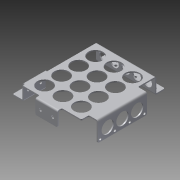
# Autodesk Inventor part: Chassis Battery Mount Part1
Saved by Autodesk Inventor 2013 (Build 170138000, 138)
## iProperties
Created: 2013-01-24
Part Number: Chassis Battery Mount Part1
Material: Aluminum 6061
Document SubType Name: Sheet Metal
Designer: Moses
Density: 2.71 g/cm^3
Sheet Metal Rule: Default
Mass: 289.922 g
Surface Area: 784.778 cm^2
Volume: 106.982 cm^3
Flat Pattern Width: 28.8793 cm
Flat Pattern Length: 29.5143 cm
Flat Pattern Area: 852.352 cm^2
Sheet Metal Width: 11.370 in
Sheet Metal Length: 11.620 in
Sheet Metal Area: 132.115 in^2
Author: Moses
Autodesk Inventor part; units mm, degrees
ref_plane "YZ Plane" through (0, 0, 0) normal (1, 0, 0) x (0, 1, 0)
ref_plane "XZ Plane" through (0, 0, 0) normal (0, 1, 0) x (-1, 0, 0)
ref_plane "XY Plane" through (0, 0, 0) normal (0, 0, 1) x (1, 0, 0)
sketch "Sketch1" plane through (0, 0, 0) normal (0, 1, 0) x (-1, 0, 0)
  line L0 (0, 0) -> (152.4, 0)
  line L1 (152.4, 0) -> (152.4, 25.4)
  line L2 (152.4, 25.4) -> (0, 25.4)
  line L3 (0, 25.4) -> (0, 0)
  line L4 (0, 12.7) -> (152.4, 12.7) construction
  circle A0 centre (12.7, 12.7) radius 3.302
  circle A1 centre (38.1, 12.7) radius 3.302
  circle A2 centre (63.5, 12.7) radius 3.302
  circle A3 centre (88.9, 12.7) radius 3.302
  circle A4 centre (114.3, 12.7) radius 3.302
  circle A5 centre (139.7, 12.7) radius 3.302
  dimension "d0" = 25.4
  dimension "d1" = 152.4
  dimension "d2" = 6.604
  dimension "d3" = 12.7
  dimension "d6" = 25.4
  dimension "d11" = 12.7
  measures "d0" distance of L2.end L0.start
  measures "d1" distance of L0.start L0.end
  measures "d2" diameter of A0
  measures "d3" distance from line of A0.centre L3
  measures "d6" distance of A0.centre A1.centre
  measures "d11" distance from line of L1 A5.centre
extrude "Plate1" add sketch "Sketch1" along normal blind 3.175
sketch "Sketch2" plane through (0, 0, 22.225) normal (0, 0, 1) x (1, 0, 0)
  line L0 (-152.4, 0) -> (0, 0)
  line L1 (0, 0) -> (0, 38.1)
  line L2 (0, 38.1) -> (-152.4, 38.1)
  line L3 (-152.4, 38.1) -> (-152.4, 0)
  constraints: 6 end point, 1 horizontal, 1 perpendicular, 1 vertical
edge flange "Flange1" height 38.1 angle 90 thickness 3.175 bend radius 1.27 thickness toward (0, 0, 1) relief straight relief width 3.175 relief depth 1.5875 edges at (-76.2, 3.175, 25.4) wall of the first edge with corners at (-152.4, 0, 22.225) (0, 0, 22.225) (0, 38.1, 22.225) (-152.4, 38.1, 22.225)
bend "Bend1"
corner "Corner1"
sketch "Sketch3" plane through (-152.4, 38.1, 25.4) normal (0, 1, 0) x (-1, 0, 0)
  line L0 (-152.4, 0) -> (0, 0)
  line L1 (0, 0) -> (0, 190.5)
  line L2 (0, 190.5) -> (-152.4, 190.5)
  line L3 (-152.4, 190.5) -> (-152.4, 0)
  constraints: 6 end point, 1 horizontal, 1 perpendicular, 1 vertical
edge flange "Flange2" height 193.675 angle 90 thickness 3.175 bend radius 1.27 thickness toward (0, 1, 0) relief straight relief width 3.175 relief depth 1.5875 edges at (-76.2, 38.1, 25.4) wall of the first edge with corners at (0, 38.1, 25.4) (-152.4, 38.1, 25.4) (-152.4, 38.1, 215.9) (0, 38.1, 215.9)
bend "Bend2"
corner "Corner2"
sketch "Sketch4" plane through (-152.4, 41.275, 215.9) normal (0, 1, 0) x (1, 0, 0)
  line L0 (0, 0) -> (0, 189.23) projected
  line L1 (152.4, 189.23) -> (152.4, 0) projected
  line L2 (-6.35, 6.35) -> (-6.35, 63.5)
  line L3 (-6.35, 63.5) -> (0, 63.5)
  line L4 (152.4, 189.23) -> (0, 189.23) projected
  line L5 (152.4, 0) -> (0, 0) projected
  circle A0 centre (28.575, 28.575) radius 19.05
  circle A1 centre (28.575, 72.6017) radius 19.05
  circle A2 centre (28.575, 116.6283) radius 19.05
  circle A3 centre (28.575, 160.655) radius 19.05
  circle A4 centre (76.2, 28.575) radius 19.05
  circle A5 centre (76.2, 72.6017) radius 19.05
  circle A6 centre (76.2, 116.6283) radius 19.05
  circle A7 centre (76.2, 160.655) radius 19.05
  circle A8 centre (123.825, 28.575) radius 19.05
  circle A9 centre (123.825, 72.6017) radius 19.05
  circle A10 centre (123.825, 116.6283) radius 19.05
  circle A11 centre (123.825, 160.655) radius 19.05
  line L6 (171.45, 19.05) -> (171.45, 146.05)
  line L7 (171.45, 146.05) -> (152.4, 146.05)
  line L8 (101.6, 0) -> (101.6, -6.35)
  line L9 (101.6, -6.35) -> (44.45, -6.35)
  line L10 (44.45, -6.35) -> (44.45, 0)
  line L11 (152.4, 19.05) -> (171.45, 19.05)
  line L12 (-6.35, 6.35) -> (0, 6.35)
  point P0 (152.4, 215.9)
  dimension "d33" = 57.15
  dimension "d35" = 6.35
  dimension "d64" = 38.1
  dimension "d65" = 28.575
  dimension "d66" = 28.575
  dimension "d69" = 44.0267
  dimension "d72" = 47.625
  dimension "d75" = 28.575
  dimension "d76" = 28.575
  dimension "d95" = 127
  dimension "d106" = 6.35
  dimension "d107" = 57.15
  dimension "d108" = 50.8
  dimension "d119" = 19.05
  dimension "d120" = 19.05
  dimension "d121" = 6.35
  dimension "d146" = 189.23
  constraints: 18 end point, 12 centre point, 6 perpendicular, 6 point on line, 2 horizontal, 2 vertical, 1 parallel, 22 other
  measures "d33" distance of L2.start L2.end
  measures "d35" distance of L2.end L3.end
  measures "d64" diameter of A0
  measures "d65" distance from line of L0 A0.centre
  measures "d66" distance from line of L5 A0.centre
  measures "d69" distance of A0.centre A1.centre
  measures "d72" distance of A0.centre A4.centre
  measures "d75" distance from line of L1 A8.centre
  measures "d76" distance from line of L4 A3.centre
  measures "d95" distance of L6.start L6.end
  measures "d106" distance of L9.end L10.end
  measures "d107" distance of L8.end L9.end
  measures "d108" distance from line of L1.end L8
  measures "d119" distance of L11.start L6.start
  measures "d120" distance from line of L1.end L11
  measures "d121" distance between parallel lines of L5 L12
  measures "d146" distance of L0.start L0.end
sheet face with bend "Face2" sketch "Sketch4" thickness 3.175 toward (0, -1, 0) bend radius 3.175 relief straight relief width 3.175 relief depth 1.5875 contours L12 L2 L3 L0 | L5 L8 L9 L10 | L1 L7 L6 L11
bend "Bend3"
sketch "Sketch5" plane through (-155.575, 41.275, 152.4) normal (-1, 0, 0) x (0, -1, 0)
  line L0 (0, 57.15) -> (0, 0)
  line L1 (0, 0) -> (41.275, 0)
  line L2 (41.275, 0) -> (41.275, 57.15)
  line L3 (41.275, 57.15) -> (0, 57.15)
  constraints: 6 end point, 1 horizontal, 1 perpendicular, 1 vertical
edge flange "Flange3" height 41.275 angle 90 thickness 3.175 bend radius 1.27 thickness toward (-1, 0, 0) relief straight relief width 3.175 relief depth 1.5875 edges at (-158.75, 38.1, 180.975) wall of the first edge with corners at (-155.575, 41.275, 209.55) (-155.575, 41.275, 152.4) (-155.575, 0, 152.4) (-155.575, 0, 209.55)
bend "Bend4"
corner "Corner3"
sketch "Sketch6" plane through (-155.575, 3.175, 209.55) normal (0, -1, 0) x (1, 0, 0)
  line L0 (0, -57.15) -> (0, 0)
  line L1 (0, 0) -> (-28.575, 0)
  line L2 (-28.575, 0) -> (-28.575, -57.15)
  line L3 (-28.575, -57.15) -> (0, -57.15)
  constraints: 6 end point, 1 horizontal, 1 perpendicular, 1 vertical
edge flange "Flange4" height 28.575 angle 90 thickness 3.175 bend radius 1.27 thickness toward (0, -1, 0) relief straight relief width 3.175 relief depth 1.5875 edges at (-158.75, 0, 180.975) wall of the first edge with corners at (-155.575, 3.175, 152.4) (-155.575, 3.175, 209.55) (-184.15, 3.175, 209.55) (-184.15, 3.175, 152.4)
bend "Bend5"
corner "Corner4"
sketch "Sketch7" plane through (-184.15, 3.175, 209.55) normal (0, 1, 0) x (1, 0, 0)
  circle A0 centre (12.7, 19.05) radius 3.302 projected
  circle A1 centre (12.7, 38.1) radius 3.302 projected
  point P0 (184.15, 209.55)
extrude "Cut1" cut sketch "Sketch7" against normal blind 3.175
fillet "Corner Round1" radius 3.175 10 edges at (-184.15, 1.5875, 209.55) (-184.15, 1.5875, 152.4) (-152.4, 1.5875, 0) (0, 1.5875, 0) (0, 39.6875, 69.85) (0, 39.6875, 196.85) (-50.8, 39.6875, 215.9) (-107.95, 39.6875, 215.9) (0, 39.6875, 215.9) (-152.4, 39.6875, 215.9)
extrude "Cut2" cut sketch "Sketch4" against normal blind 3.175 contours A0 | A1 | A2 | A3 | A4 | A5 | A6 | A7 | A8 | A9 | A10 | A11
sketch "Sketch8" plane through (0, 4.445, 22.225) normal (0, 0, -1) x (-1, 0, 0)
  line L0 (0, 32.385) -> (0, 0) projected
  line L1 (152.4, 32.385) -> (152.4, 0) projected
  line L2 (0, 16.1925) -> (152.4, 16.1925) construction
  circle A0 centre (19.05, 16.1925) radius 11.1125
  circle A1 centre (47.625, 16.1925) radius 11.1125
  circle A2 centre (76.2, 16.1925) radius 11.1125
  circle A3 centre (104.775, 16.1925) radius 11.1125
  circle A4 centre (133.35, 16.1925) radius 11.1125
  point P0 (0, -4.445)
  dimension "d79" = 22.225
  dimension "d83" = 19.05
  dimension "d84" = 152.4
  dimension "d87" = 28.575
  constraints: 5 centre point, 2 end point, 2 midpoint, 1 horizontal, 1 point on line, 8 other
  measures "d79" diameter of A0
  measures "d83" distance from line of A0.centre L0
  measures "d84" distance of L1.start L0.start
  measures "d87" distance of A0.centre A1.centre
extrude "Cut3" cut sketch "Sketch8" against normal blind 3.175
sketch "Sketch9" plane through (20.32, 36.83, 196.85) normal (1, 0, 0) x (0, 1, 0)
  line L0 (0, -127) -> (0, 0)
  line L1 (0, 0) -> (-46.355, 0)
  line L2 (-46.355, 0) -> (-46.355, -127)
  line L3 (-46.355, -127) -> (0, -127)
  constraints: 6 end point, 1 horizontal, 1 perpendicular, 1 vertical
edge flange "Flange5" height 50.8 angle 90 thickness 3.175 bend radius 1.27 thickness toward (1, 0, 0) relief straight relief width 3.175 relief depth 1.5875 edges at (19.05, 38.1, 133.35) wall of the first edge with corners at (20.32, 36.83, 69.85) (20.32, 36.83, 196.85) (20.32, -9.525, 196.85) (20.32, -9.525, 69.85)
bend "Bend6"
corner "Corner5"
sketch "Sketch10" plane through (-107.95, 36.83, 223.52) normal (0, 0, 1) x (1, 0, 0)
  line L0 (57.15, 0) -> (0, 0)
  line L1 (0, 0) -> (0, -33.655)
  line L2 (0, -33.655) -> (57.15, -33.655)
  line L3 (57.15, -33.655) -> (57.15, 0)
  constraints: 6 end point, 1 horizontal, 1 perpendicular, 1 vertical
edge flange "Flange6" height 38.1 angle 90 thickness 3.175 bend radius 1.27 thickness toward (0, 0, 1) relief straight relief width 3.175 relief depth 1.5875 edges at (-79.375, 38.1, 222.25) wall of the first edge with corners at (-50.8, 36.83, 223.52) (-107.95, 36.83, 223.52) (-107.95, 3.175, 223.52) (-50.8, 3.175, 223.52)
bend "Bend7"
corner "Corner6"
sketch "Sketch11" plane through (23.495, -9.525, 196.85) normal (1, 0, 0) x (0, 0, -1)
  line L0 (0, 0) -> (0, 46.355) projected
  line L1 (127, 0) -> (0, 0) projected
  line L2 (127, 46.355) -> (127, 0) projected
  line L3 (0, 23.1775) -> (127, 23.1775) construction
  circle A0 centre (25.4, 23.1775) radius 15.875
  circle A1 centre (63.5, 23.1775) radius 15.875
  circle A2 centre (101.6, 23.1775) radius 15.875
  line L4 (0, 6.35) -> (127, 6.35) construction
  circle A3 centre (6.35, 6.35) radius 3.302
  circle A4 centre (44.45, 6.35) radius 3.302
  circle A5 centre (82.55, 6.35) radius 3.302
  circle A6 centre (120.65, 6.35) radius 3.302
  point P0 (196.85, 9.525)
  dimension "d122" = 127
  dimension "d123" = 31.75
  dimension "d124" = 25.4
  dimension "d127" = 38.1
  dimension "d132" = 25.4
  dimension "d133" = 6.35
  dimension "d134" = 6.604
  dimension "d135" = 6.35
  dimension "d138" = 38.1
  dimension "d143" = 6.35
  constraints: 7 centre point, 4 end point, 4 point on line, 2 horizontal, 2 midpoint, 1 perpendicular, 10 other
  measures "d122" distance of L2.start L0.end
  measures "d123" diameter of A0
  measures "d124" distance from line of A0.centre L0
  measures "d127" distance of A0.centre A1.centre
  measures "d132" distance from line of L2 A2.centre
  measures "d133" distance between parallel lines of L1 L4
  measures "d134" diameter of A3
  measures "d135" distance from line of A3.centre L0
  measures "d138" distance of A3.centre A4.centre
  measures "d143" distance from line of L2 A6.centre
extrude "Cut4" cut sketch "Sketch11" against normal blind 3.175
sketch "Sketch12" plane through (-158.75, 36.83, 152.4) normal (-1, 0, 0) x (0, 0, 1)
  line L0 (57.15, 0) -> (57.15, -32.385) projected
  line L1 (0, -32.385) -> (0, 0) projected
  line L2 (0, -16.1925) -> (57.15, -16.1925) construction
  circle A0 centre (12.7, -16.1925) radius 3.302
  circle A1 centre (44.45, -16.1925) radius 3.302
  point P0 (-152.4, -36.83)
  dimension "d147" = 6.604
  dimension "d149" = 12.7
  dimension "d150" = 12.7
  constraints: 2 centre point, 2 end point, 2 midpoint, 2 point on line, 1 equal radius
  measures "d147" diameter of A1
  measures "d149" distance from line of L0 A1.centre
  measures "d150" distance from line of L1 A0.centre
extrude "Cut5" cut sketch "Sketch12" against normal blind 3.175
sketch "Sketch13" plane through (-107.95, 3.175, 226.695) normal (0, 0, 1) x (1, 0, 0)
  line L0 (0, 0) -> (0, 33.655) projected
  line L1 (57.15, 33.655) -> (57.15, 0) projected
  line L2 (0, 16.8275) -> (57.15, 16.8275) construction
  circle A0 centre (12.7, 16.8275) radius 3.302
  circle A1 centre (44.45, 16.8275) radius 3.302
  point P0 (107.95, -3.175)
  dimension "d153" = 6.604
  dimension "d155" = 12.7
  dimension "d156" = 12.7
  constraints: 2 centre point, 2 end point, 2 midpoint, 2 point on line, 1 equal radius
  measures "d153" diameter of A1
  measures "d155" distance from line of L1 A1.centre
  measures "d156" distance from line of L0 A0.centre
extrude "Cut6" cut sketch "Sketch13" against normal blind 3.175
fillet "Corner Round2" radius 3.175 4 edges at (-50.8, 3.175, 225.1075) (-107.95, 3.175, 225.1075) (21.9075, -9.525, 196.85) (21.9075, -9.525, 69.85)
equation "\"d69\" = -0.666667 * d66 + 0.333333 * d146"
equation "\"d61\" = Thickness"
equation "\"d77\" = Thickness"
equation "\"d87\" = -0.5 * d83 + 0.25 * d84"
equation "\"d92\" = Thickness"
equation "\"d127\" = -d124 + 0.5 * d122"
equation "\"d144\" = Thickness"
equation "\"d13\" = BendReliefWidth"
equation "\"d14\" = BendReliefDepth"
equation "\"d15\" = MinimumRemnant"
equation "\"d16\" = BendRadius"
equation "\"d20\" = CornerReliefSize"
equation "\"d21\" = GapSize"
equation "\"d22\" = JacobiRadiusSize"
equation "\"d23\" = BendReliefWidth"
equation "\"d24\" = BendReliefDepth"
equation "\"d25\" = MinimumRemnant"
equation "\"d26\" = BendRadius"
equation "\"d30\" = CornerReliefSize"
equation "\"d31\" = GapSize"
equation "\"d32\" = JacobiRadiusSize"
equation "\"d36\" = BendRadius"
equation "\"d37\" = BendReliefWidth"
equation "\"d39\" = MinimumRemnant"
equation "\"d38\" = BendReliefDepth"
equation "\"d40\" = BendRadius"
equation "\"d41\" = BendReliefWidth"
equation "\"d42\" = BendReliefDepth"
equation "\"d43\" = MinimumRemnant"
equation "\"d44\" = BendRadius"
equation "\"d48\" = CornerReliefSize"
equation "\"d49\" = GapSize"
equation "\"d50\" = JacobiRadiusSize"
equation "\"d51\" = BendReliefWidth"
equation "\"d52\" = BendReliefDepth"
equation "\"d53\" = MinimumRemnant"
equation "\"d54\" = BendRadius"
equation "\"d58\" = CornerReliefSize"
equation "\"d59\" = GapSize"
equation "\"d60\" = JacobiRadiusSize"
equation "\"d96\" = BendReliefWidth"
equation "\"d97\" = BendReliefDepth"
equation "\"d98\" = MinimumRemnant"
equation "\"d99\" = BendRadius"
equation "\"d103\" = CornerReliefSize"
equation "\"d104\" = GapSize"
equation "\"d105\" = JacobiRadiusSize"
equation "\"d109\" = BendReliefWidth"
equation "\"d110\" = BendReliefDepth"
equation "\"d111\" = MinimumRemnant"
equation "\"d112\" = BendRadius"
equation "\"d116\" = CornerReliefSize"
equation "\"d117\" = GapSize"
equation "\"d118\" = JacobiRadiusSize"
equation "\"BendRadius\" = Thickness"
equation "\"BendReliefWidth\" = Thickness"
equation "\"BendReliefDepth\" = 0.5 * Thickness"
equation "\"CornerReliefSize\" = 4 * Thickness"
equation "\"MinimumRemnant\" = 2 * Thickness"
equation "\"TransitionRadius\" = BendRadius"
equation "\"JacobiRadiusSize\" = BendRadius"
equation "\"GapSize\" = Thickness"
equation "\"d12\" = BendRadius"
equation "\"Thickness\" = 3.175"
body "Solid1"
